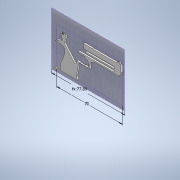
# Autodesk Inventor part: sheetmettaal_2
Saved by Autodesk Inventor 2022 (Build 260153000, 153)
## iProperties
Created: 2022-05-17
Part Number: sheetmettaal_2
Material: Generic
Document SubType Name: Sheet Metal
Designer: joshn
Density: 1 g/cm^3
Sheet Metal Rule: Default
Appearance: Default
Author: joshn
Autodesk Inventor part; units mm, degrees
ref_plane "YZ Plane" through (0, 0, 0) normal (1, 0, 0) x (0, 1, 0)
ref_plane "XZ Plane" through (0, 0, 0) normal (0, 1, 0) x (-1, 0, 0)
ref_plane "XY Plane" through (0, 0, 0) normal (0, 0, 1) x (1, 0, 0)
sketch "Sketch6" plane through (0, 0, 0) normal (0, 0, 1) x (1, 0, 0)
  line L0 (-5.6746, 52.8838) -> (72.2159, 52.8838) construction
  line L1 (72.2159, 52.8838) -> (72.2159, -3.6669) construction
  line L2 (72.2159, -3.6669) -> (-5.6746, -3.6669) construction
  line L3 (-5.6746, -3.6669) -> (-5.6746, 52.8838) construction
  point P0 (0, 0)
  dimension "d101" = 77.8905
  constraints: 2 other
  measures "d101" distance of L1.end L2.end
sketch "Sketch5" plane through (0, 0, 0) normal (0, 0, 1) x (1, 0, 0)
  line L0 (-5.6746, 50.6241) -> (72.2159, 50.6241) construction
  line L1 (72.2159, 50.6241) -> (72.2159, -5.9265) construction
  line L2 (72.2159, -5.9265) -> (-5.6746, -5.9265) construction
  line L3 (-5.6746, -5.9265) -> (-5.6746, 50.6241) construction
  point P0 (0, 0)
  dimension "d87" = 5.6746
  dimension "d93" = 5.9265
  dimension "d94" = 77.8905
  constraints: 1 vertical, 2 other
  measures "d87" horizontal distance of L2.end point (0, 0)
  measures "d93" vertical distance of L2.end point (0, 0)
  measures "d94" distance of L1.end L2.end
sketch "Sketch2" plane through (0, 0, 0) normal (0, 0, 1) x (1, 0, 0)
  line L0 (-0.0649, 40.1311) -> (69.9351, 40.1311) construction
  line L1 (69.9351, 40.1311) -> (69.9351, 0.2211) construction
  line L2 (69.9351, 0.2211) -> (-0.0649, 0.2211) construction
  line L3 (-0.0649, 0.2211) -> (-0.0649, 40.1311) construction
  point P0 (0, 0)
  dimension "d25" = 70
  constraints: 1 vertical, 2 other
  measures "d25" distance of L1.end L2.end
sketch "Sketch4" plane through (0, 0, 0) normal (0, 0, 1) x (1, 0, 0)
  line L0 (19.5619, 38.7676) -> (30.0991, 38.7676)
  line L1 (30.0991, 38.7676) -> (30.0991, 38.3986)
  line L2 (30.0991, 38.3986) -> (39.1755, 38.3986)
  line L3 (40.1184, 38.0799) -> (64.6623, 38.0799)
  line L4 (65.258, 38.3986) -> (69.8165, 38.3986)
  line L5 (69.8165, 38.3986) -> (69.8165, 31.2615)
  line L6 (69.8165, 31.2615) -> (67.9887, 26.9086)
  line L7 (67.9887, 26.9086) -> (42.9206, 26.9086)
  arc A0 (39.1755, 38.3986) -> (40.1184, 38.0799) centre (40.1184, 39.634) ccw
  arc A1 (64.6623, 38.0799) -> (65.258, 38.3986) centre (64.6623, 38.7959) ccw
  line L8 (14.858, 37.6857) -> (17.3096, 37.6857)
  arc A2 (17.3096, 37.6857) -> (19.5619, 38.7676) centre (17.3096, 40.571) ccw
  line L9 (14.858, 37.6857) -> (15.3567, 36.9178)
  line L10 (15.3567, 36.9178) -> (12.6859, 36.9178)
  line L11 (12.6859, 36.9178) -> (13.1845, 37.6857)
  line L12 (13.1845, 37.6857) -> (11.7392, 37.6857)
  line L13 (11.7392, 37.6857) -> (8.1785, 34.1028)
  line L14 (8.1785, 34.1028) -> (7.059, 29.9087)
  line L15 (14.0213, 36.9178) -> (14.0213, 38.1679) construction
  arc A3 (5.437, 28.5166) -> (7.059, 29.9087) centre (5.232, 30.3964) ccw
  arc A4 (5.437, 28.5166) -> (0.0997, 26.2441) centre (6.5221, 18.5643) ccw
  arc A5 (0.0997, 26.2441) -> (0.2271, 25.8932) centre (0.2271, 26.0917) ccw
  line L16 (0.2271, 25.8932) -> (5.4711, 25.8932)
  arc A6 (10.0514, 19.7373) -> (5.4711, 25.8932) centre (5.4711, 21.1112) ccw
  line L17 (10.0514, 19.7373) -> (8.5865, 14.854)
  arc A7 (6.2353, 9.2686) -> (5.3348, 5.3158) centre (12.6207, 5.735) ccw
  arc A8 (6.2353, 9.2686) -> (8.5865, 14.854) centre (-18.5877, 23.0055) ccw
  line L18 (5.3348, 5.3158) -> (5.5341, 1.852)
  line L19 (5.5341, 1.852) -> (6.8626, 1.2503)
  line L20 (6.8626, 1.2503) -> (23.5585, 1.2503)
  line L21 (23.5585, 1.2503) -> (22.5575, 3.7645)
  arc A9 (22.4158, 5.1753) -> (22.5575, 3.7645) centre (24.951, 4.7174) ccw
  line L22 (22.4158, 5.1753) -> (24.5105, 16.2688)
  arc A10 (27.2251, 18.1204) -> (24.5105, 16.2688) centre (26.7933, 15.8377) ccw
  line L23 (27.2251, 18.1204) -> (28.3169, 17.7569)
  line L24 (28.3169, 17.7569) -> (36.2548, 17.7569)
  arc A11 (36.2548, 17.7569) -> (36.6826, 18.3442) centre (36.2548, 18.2063) ccw
  arc A12 (42.9206, 26.9086) -> (36.6826, 18.3442) centre (42.9206, 20.3546) ccw
  line L25 (29.5614, 25.8932) -> (31.5766, 25.8932)
  arc A13 (35.4302, 22.0395) -> (31.5766, 25.8932) centre (31.5766, 22.0395) ccw
  line L26 (35.4302, 22.0395) -> (35.4302, 19.8111)
  arc A14 (27.9975, 25.1393) -> (26.6981, 19.4379) centre (29.1407, 21.8799) ccw
  arc A15 (26.6981, 19.4379) -> (28.9176, 18.5344) centre (28.8794, 21.6187) ccw
  arc A16 (27.9975, 25.1393) -> (29.1072, 25.7392) centre (26.6723, 28.9172) ccw
  arc A17 (29.5614, 25.8932) -> (29.1072, 25.7392) centre (29.5614, 25.1464) ccw
  line L27 (28.8763, 18.5342) -> (34.1533, 18.5342)
  arc A18 (34.1533, 18.5342) -> (35.4302, 19.8111) centre (34.1533, 19.8111) ccw
  line L28 (8.1785, 34.1028) -> (27.2251, 18.1204) construction
  line L29 (9.5846, 28.3084) -> (62.5732, 28.3084)
  line L30 (62.5732, 33.5244) -> (31.484, 33.5244)
  arc A19 (30.0991, 34.9092) -> (31.484, 33.5244) centre (31.484, 34.9092) ccw
  line L31 (30.0991, 34.9092) -> (30.0991, 38.3986)
  line L32 (9.5846, 28.3084) -> (12.1362, 37.6857)
  line L33 (32.1812, 31.5548) -> (62.5732, 31.5548)
  line L34 (62.5732, 30.278) -> (32.1812, 30.278)
  line L35 (32.1812, 30.278) -> (32.1812, 31.5548)
  line L36 (62.5732, 28.3084) -> (62.5732, 30.278)
  line L37 (62.5732, 31.5548) -> (62.5732, 33.5244)
  point P0 (0, 0)
  point P1 (30.569, 25.8932)
  constraints: 76 end point, 41 point on circle, 27 tangent, 20 centre point, 19 horizontal, 5 perpendicular, 4 parallel, 3 vertical, 2 collinear, 2 midpoint, 1 point on line, 1 other
sketch "Sketch7" plane through (0, 0, 0) normal (0, 0, 1) x (1, 0, 0)
  line L0 (19.5619, 38.7676) -> (30.0991, 38.7676)
  line L1 (30.0991, 38.7676) -> (30.0991, 38.3986)
  line L2 (30.0991, 38.3986) -> (39.1755, 38.3986)
  line L3 (40.1184, 38.0799) -> (64.6623, 38.0799)
  line L4 (65.258, 38.3986) -> (69.8165, 38.3986)
  line L5 (69.8165, 38.3986) -> (69.8165, 31.2615)
  line L6 (69.8165, 31.2615) -> (67.9887, 26.9086)
  line L7 (67.9887, 26.9086) -> (42.9206, 26.9086)
  arc A0 (39.1755, 38.3986) -> (40.1184, 38.0799) centre (40.1184, 39.634) ccw
  arc A1 (64.6623, 38.0799) -> (65.258, 38.3986) centre (64.6623, 38.7959) ccw
  line L8 (14.858, 37.6857) -> (17.3096, 37.6857)
  arc A2 (17.3096, 37.6857) -> (19.5619, 38.7676) centre (17.3096, 40.571) ccw
  line L9 (14.858, 37.6857) -> (15.3567, 36.9178)
  line L10 (15.3567, 36.9178) -> (12.6859, 36.9178)
  line L11 (12.6859, 36.9178) -> (13.1845, 37.6857)
  line L12 (13.1845, 37.6857) -> (11.7392, 37.6857)
  line L13 (11.7392, 37.6857) -> (8.1785, 34.1028)
  line L14 (8.1785, 34.1028) -> (7.059, 29.9087)
  line L15 (14.0213, 36.9178) -> (14.0213, 38.1679) construction
  arc A3 (5.437, 28.5166) -> (7.059, 29.9087) centre (5.232, 30.3964) ccw
  arc A4 (5.437, 28.5166) -> (0.0997, 26.2441) centre (6.5221, 18.5643) ccw
  arc A5 (0.0997, 26.2441) -> (0.2271, 25.8932) centre (0.2271, 26.0917) ccw
  line L16 (0.2271, 25.8932) -> (5.4711, 25.8932)
  arc A6 (10.0514, 19.7373) -> (5.4711, 25.8932) centre (5.4711, 21.1112) ccw
  line L17 (10.0514, 19.7373) -> (8.5865, 14.854)
  arc A7 (6.2353, 9.2686) -> (5.3348, 5.3158) centre (12.6207, 5.735) ccw
  arc A8 (6.2353, 9.2686) -> (8.5865, 14.854) centre (-18.5877, 23.0055) ccw
  line L18 (5.3348, 5.3158) -> (5.5341, 1.852)
  line L19 (5.5341, 1.852) -> (6.8626, 1.2503)
  line L20 (6.8626, 1.2503) -> (23.5585, 1.2503)
  line L21 (23.5585, 1.2503) -> (22.5575, 3.7645)
  arc A9 (22.4158, 5.1753) -> (22.5575, 3.7645) centre (24.951, 4.7174) ccw
  line L22 (22.4158, 5.1753) -> (24.5105, 16.2688)
  arc A10 (27.2251, 18.1204) -> (24.5105, 16.2688) centre (26.7933, 15.8377) ccw
  line L23 (27.2251, 18.1204) -> (28.3169, 17.7569)
  line L24 (28.3169, 17.7569) -> (36.2548, 17.7569)
  arc A11 (36.2548, 17.7569) -> (36.6826, 18.3442) centre (36.2548, 18.2063) ccw
  arc A12 (42.9206, 26.9086) -> (36.6826, 18.3442) centre (42.9206, 20.3546) ccw
  line L25 (29.5614, 25.8932) -> (31.5766, 25.8932)
  arc A13 (35.4302, 22.0395) -> (31.5766, 25.8932) centre (31.5766, 22.0395) ccw
  line L26 (35.4302, 22.0395) -> (35.4302, 19.8111)
  arc A14 (27.9975, 25.1393) -> (26.6981, 19.4379) centre (29.1407, 21.8799) ccw
  arc A15 (26.6981, 19.4379) -> (28.9176, 18.5344) centre (28.8794, 21.6187) ccw
  arc A16 (27.9975, 25.1393) -> (29.1072, 25.7392) centre (26.6723, 28.9172) ccw
  arc A17 (29.5614, 25.8932) -> (29.1072, 25.7392) centre (29.5614, 25.1464) ccw
  line L27 (28.8763, 18.5342) -> (34.1533, 18.5342)
  arc A18 (34.1533, 18.5342) -> (35.4302, 19.8111) centre (34.1533, 19.8111) ccw
  line L28 (8.1785, 34.1028) -> (27.2251, 18.1204) construction
  line L29 (9.5846, 28.3084) -> (62.5732, 28.3084)
  line L30 (62.5732, 33.5244) -> (31.484, 33.5244)
  arc A19 (30.0991, 34.9092) -> (31.484, 33.5244) centre (31.484, 34.9092) ccw
  line L31 (30.0991, 34.9092) -> (30.0991, 38.3986)
  line L32 (9.5846, 28.3084) -> (12.1362, 37.6857)
  line L33 (32.1812, 31.5548) -> (62.5732, 31.5548)
  line L34 (62.5732, 30.278) -> (32.1812, 30.278)
  line L35 (32.1812, 30.278) -> (32.1812, 31.5548)
  line L36 (62.5732, 28.3084) -> (62.5732, 30.278)
  line L37 (62.5732, 31.5548) -> (62.5732, 33.5244)
  line L38 (9.5846, 28.3084) -> (19.9132, 15.7819)
  arc A20 (19.9132, 15.7819) -> (22.2081, 16.2806) centre (20.9323, 16.6221) ccw
  line L39 (22.8832, 18.8031) -> (22.2081, 16.2806)
  line L40 (31.0105, 18.5342) -> (31.0105, 17.7569) construction
  line L41 (31.0105, 18.1455) -> (28.6028, 18.1717)
  arc A21 (26.6981, 18.8031) -> (28.6028, 18.1717) centre (28.6386, 21.4681) ccw
  line L42 (26.6981, 18.8031) -> (22.8832, 18.8031)
  line L43 (31.0105, 18.1455) -> (31.0105, 18.5342)
  line L44 (31.0105, 18.5342) -> (31.0105, 25.8932) construction
  line L45 (24.5105, 28.3084) -> (23.9563, 27.1008)
  line L46 (23.9563, 27.1008) -> (31.0105, 27.1008)
  line L47 (31.0105, 27.1008) -> (31.0105, 25.8932)
  line L48 (31.0105, 27.1008) -> (31.0105, 28.3084) construction
  line L49 (65.4825, 38.3986) -> (65.4825, 38.8805)
  line L50 (65.4825, 38.8805) -> (67.4545, 40.0926)
  line L51 (67.4545, 40.0926) -> (67.8962, 40.0926)
  arc A22 (68.6185, 39.3704) -> (67.8962, 40.0926) centre (67.8962, 39.3704) ccw
  line L52 (68.6185, 39.3704) -> (68.6185, 38.3986)
  point P0 (0, 0)
  point P1 (0, 0)
  point P2 (30.569, 25.8932)
extrude "Plate4" add sketch "Sketch7" along normal blind 1.5 contours L2 A0 L3 A1 L4 L5 L6 L7 A12 A11 L24 L23 A10 L22 A9 L21 L20 L19 L18 A7 A8 L17 A6 L16 A5 A4 A3 L14 L13 L12 L32 L38 A20 L39 L42 A21 L41 L43 L27 A18 L26 A13 L25 L47 L46 L45 L29 L36 L34 L35 L33 L37 L30 A19 L31 | L49 L50 L51 A22 L52 L4
sketch "Sketch8" plane through (0, 0, 1.5) normal (0, 0, 1) x (1, 0, 0)
  line L0 (8.1785, 34.1028) -> (7.059, 29.9087) construction
  arc A0 (7.059, 29.9087) -> (5.336, 34.6737) centre (2.7728, 31.0528) ccw
  line L1 (7.059, 29.9087) -> (8.1785, 34.1028)
  arc A1 (5.8207, 36.0777) -> (5.336, 34.6737) centre (5.783, 35.3051) ccw
  line L2 (5.8207, 36.0777) -> (6.4315, 36.0478)
  line L3 (6.4315, 36.0478) -> (6.5683, 35.7333)
  line L4 (6.5683, 35.7333) -> (6.7449, 35.9935)
  line L5 (6.7449, 35.9935) -> (6.8817, 35.679)
  line L6 (6.8817, 35.679) -> (7.0584, 35.9392)
  line L7 (7.0584, 35.9392) -> (7.1662, 35.6297)
  line L8 (7.1662, 35.6297) -> (7.3428, 35.89)
  line L9 (7.3428, 35.89) -> (7.4931, 35.5731)
  line L10 (7.4931, 35.5731) -> (7.6697, 35.8333)
  line L11 (7.6697, 35.8333) -> (7.8065, 35.5188)
  line L12 (7.8065, 35.5188) -> (7.9831, 35.779)
  line L13 (7.9831, 35.779) -> (8.1199, 35.4645)
  line L14 (8.1199, 35.4645) -> (8.2965, 35.7248)
  line L15 (8.2965, 35.7248) -> (8.4333, 35.4102)
  line L16 (8.4333, 35.4102) -> (8.6099, 35.6705)
  line L17 (6.4315, 36.0478) -> (8.6099, 35.6705) construction
  line L18 (6.5683, 35.7333) -> (8.4333, 35.4102) construction
  line L19 (8.1785, 34.1028) -> (11.7392, 37.6857)
  arc A2 (9.571, 35.504) -> (8.6099, 35.6705) centre (8.9541, 34.8004) ccw
  point P0 (0, 0)
sheet face with bend "Face5" sketch "Sketch8" thickness 1.5 toward (0, 0, -1) bend radius 1.5
bend "Bend1"
sketch "Sketch9" plane through (0, 0, 0) normal (0, 0, -1) x (-1, 0, 0)
  line L0 (-11.7034, 36.0951) -> (-12.1362, 37.6857) projected
  line L1 (-10.1584, 36.0951) -> (-11.7034, 36.0951) projected
  line L2 (-11.7392, 37.6857) -> (-10.1584, 36.0951) projected
  line L3 (-12.1362, 37.6857) -> (-11.7392, 37.6857) projected
  point P0 (0, 0)
extrude "Cut1" cut sketch "Sketch9" against normal blind 1.5
equation "\"d101\" = d94"
equation "\"d130\" = Thickness"
equation "\"d121\" = Thickness"
equation "\"d125\" = BendRadius"
equation "\"d126\" = BendReliefWidth"
equation "\"d128\" = MinimumRemnant"
equation "\"d127\" = BendReliefDepth"
equation "\"d129\" = TransitionRadius"
equation "\"BendRadius\" = Thickness"
equation "\"BendReliefWidth\" = Thickness"
equation "\"BendReliefDepth\" = 0.5 * Thickness"
equation "\"CornerReliefSize\" = 4 * Thickness"
equation "\"MinimumRemnant\" = 2 * Thickness"
equation "\"TransitionRadius\" = BendRadius"
equation "\"JacobiRadiusSize\" = BendRadius"
equation "\"GapSize\" = Thickness"
equation "\"Thickness\" = 1.5"
body "Solid4"
